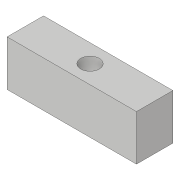
# Autodesk Inventor part: Lidar Holder 1
Saved by Autodesk Inventor 2018.3 (Build 223284000, 284)
## iProperties
Created: 2018-11-06
Part Number: Lidar Holder 1
Material: Generic
Document SubType Name: Modeling
Designer: aye06091
Mass: 68.5331 g
Surface Area: 129.478 cm^2
Volume: 68.5331 cm^3
Density: 1 g/cm^3
Appearance: Default
Author: aye06091
Autodesk Inventor part; units mm, degrees
ref_plane "YZ Plane" through (0, 0, 0) normal (1, 0, 0) x (0, 1, 0)
ref_plane "XZ Plane" through (0, 0, 0) normal (0, 1, 0) x (-1, 0, 0)
ref_plane "XY Plane" through (0, 0, 0) normal (0, 0, 1) x (1, 0, 0)
sketch "Sketch1" plane through (0, 0, 0) normal (0, 0, 1) x (1, 0, 0)
  line L0 (0, 0) -> (-90.17, 0)
  line L1 (-90.17, 0) -> (-90.17, 31.75)
  line L2 (-90.17, 31.75) -> (0, 31.75)
  line L3 (0, 31.75) -> (0, 0)
  dimension "d0" = 90.17
  dimension "d1" = 31.75
  constraints: 8 end point, 2 parallel, 1 horizontal, 1 perpendicular
  measures "d0" distance of L1.end L2.end
  measures "d1" distance of L2.end L0.start
extrude "Extrusion1" add sketch "Sketch1" against normal blind 25.4
sketch "Sketch2" plane through (-90.17, 31.75, 0) normal (0, 1, 0) x (1, 0, 0)
  line L0 (0, 0) -> (90.17, 0) projected
  line L1 (90.17, 0) -> (90.17, 25.4) projected
  line L2 (0, 25.4) -> (90.17, 25.4) projected
  line L3 (0, 0) -> (0, 25.4) projected
  line L4 (90.17, 0) -> (52.07, 0)
  line L5 (52.07, 0) -> (52.07, 25.4)
  line L6 (52.07, 25.4) -> (90.17, 25.4)
  line L7 (90.17, 25.4) -> (90.17, 0)
  line L8 (0, 0) -> (0, 25.4) projected
  line L9 (0, 0) -> (38.1, 0)
  line L10 (38.1, 0) -> (38.1, 25.4)
  line L11 (38.1, 25.4) -> (0, 25.4)
  line L12 (0, 25.4) -> (0, 0)
  line L13 (38.1, 6.223) -> (52.07, 6.223)
  line L14 (52.07, 6.223) -> (52.07, 19.177)
  line L15 (52.07, 19.177) -> (38.1, 19.177)
  line L16 (38.1, 19.177) -> (38.1, 6.223)
  circle A0 centre (45.085, 12.7) radius 6.477
  dimension "d4" = 38.1
  dimension "d5" = 38.1
  dimension "d6" = 6.223
  dimension "d7" = 6.223
  dimension "d8" = 6.477
  dimension "d10" = 6.985
  dimension "d11" = 6.985
  dimension "d12" = 12.954
  constraints: 24 end point, 6 parallel, 4 point on line, 3 horizontal, 3 perpendicular, 1 centre point, 1 coincident
  measures "d4" distance between parallel lines of L10 L3
  measures "d5" distance between parallel lines of L1 L5
  measures "d6" distance between parallel lines of L0 L13
  measures "d7" distance between parallel lines of L2 L15
  measures "d8" distance from line of L13 point (45.085, 12.7)
  measures "d10" distance from line of L10 point (45.085, 12.7)
  measures "d11" distance from line of L14 point (45.085, 12.7)
  measures "d12" diameter of A0
extrude "Extrusion2" cut sketch "Sketch2" against normal blind 76.2 contours A0
body "Solid1"
